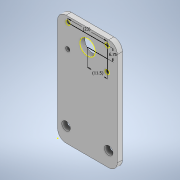
# Autodesk Inventor part: 5
Saved by Autodesk Inventor 2021 (Build 250183000, 183)
## iProperties
Created: 2021-03-30
Part Number: 5
Material: Genérico
Document SubType Name: Modeling
Designer: diego
Density: 1 g/cm^3
Appearance: Valor por defecto
Author: diego
Autodesk Inventor part; units mm, degrees
ref_plane "YZ Plane" through (0, 0, 0) normal (1, 0, 0) x (0, 1, 0)
ref_plane "XZ Plane" through (0, 0, 0) normal (0, 1, 0) x (-1, 0, 0)
ref_plane "XY Plane" through (0, 0, 0) normal (0, 0, 1) x (1, 0, 0)
sketch "Boceto1" plane through (0, 0, 0) normal (0, 0, 1) x (1, 0, 0)
  line L0 (5, 0) -> (30, 0)
  line L1 (35, 5) -> (35, 60)
  line L2 (30, 65) -> (5, 65)
  line L3 (0, 60) -> (0, 5)
  arc A0 (5, 65) -> (0, 60) centre (5, 60) ccw
  arc A1 (35, 60) -> (30, 65) centre (30, 60) ccw
  arc A2 (0, 5) -> (5, 0) centre (5, 5) ccw
  arc A3 (30, 0) -> (35, 5) centre (30, 5) ccw
  circle A4 centre (17.5, 55) radius 4.5
  circle A5 centre (29, 48.25) radius 1.25
  circle A6 centre (29, 61.75) radius 1.25
  circle A7 centre (6, 61.75) radius 1.25
  circle A8 centre (6, 48.25) radius 1.25
  circle A9 centre (5, 8.75) radius 2.5
  circle A10 centre (30, 8.75) radius 2.5
  point P0 (0, 0)
  constraints: 11 centre point, 8 end point, 8 point on circle, 8 tangent, 3 equal radius, 3 perpendicular, 2 point on line, 1 horizontal
extrude "Extrusión1" add sketch "Boceto1" along normal blind 3
sketch "Boceto2" plane through (0, 0, 3) normal (0, 0, 1) x (1, 0, 0)
  circle A0 centre (17.5, 55) radius 4.5 projected
  circle A1 centre (29, 48.25) radius 1.25 projected
  line L0 (29, 48.25) -> (29, 55)
  circle A2 centre (29, 61.75) radius 1.25 projected
  line L1 (29, 55) -> (29, 61.75)
  circle A3 centre (6, 61.75) radius 1.25 projected
  line L2 (29, 61.75) -> (6, 61.75)
  line L3 (17.5, 55) -> (29, 55)
  point P0 (0, 0)
  dimension "d20" = 23
  dimension "d21" = 6.75
  dimension "d22" = 11.5
  constraints: 8 end point, 2 vertical, 1 perpendicular
  measures "d20" distance of L1.end L2.end
  measures "d21" distance of L0.end L1.end
  measures "d22" distance of L3.start L0.end
